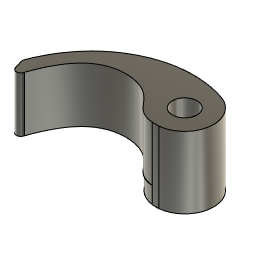
BarrelRatchet v3 (Autodesk Fusion 360 design; units mm, degrees)
Autodesk Fusion 360 part; units mm, degrees
sketch "base" plane through (0, 0, 0) normal (0, 0, 1) x (1, 0, 0)
  circle A0 centre (8.663, 2.8659) radius 2.25
  circle A1 centre (8.663, 2.8659) radius 5.25
  spline S0 degree 5 poles (-11.5756, -6.3241) (-11.5419, -6.2133) (-11.4706, -5.9871) (-11.3516, -5.634) (-11.1692, -5.1354) (-10.9008, -4.4671) (-10.591, -3.7572) (-10.2374, -3.0131) (-9.8371, -2.2479) (-9.3859, -1.4787) (-8.8802, -0.7244) (-8.3164, -0.0047) (-7.6922, 0.6618) (-7.007, 1.2599) (-6.2619, 1.777) (-5.4599, 2.2034) (-4.6063, 2.5325) (-3.7086, 2.7602) (-2.7767, 2.8854) (-1.823, 2.9086) (-0.8622, 2.8297) (0.0889, 2.6468) (1.0114, 2.3552) (1.8835, 1.9433) (2.6869, 1.4021) (3.4132, 0.7352) (4.0764, -0.0226) (4.711, -0.8083) (5.4062, -1.479) (6.2073, -1.9622) (7.1161, -2.254) (7.915, -2.3562) (8.5435, -2.3764) (8.9737, -2.3675) (9.1917, -2.3574) knots 0 0 0 0 0 0 0.033333 0.066667 0.1 0.133333 0.166667 0.2 0.233333 0.266667 0.3 0.333333 0.366667 0.4 0.433333 0.466667 0.5 0.533333 0.566667 0.6 0.633333 0.666667 0.7 0.733333 0.766667 0.8 0.833333 0.866667 0.9 0.933333 0.966667 1 1 1 1 1 1
  line L0 (2.9298, 1.2447) -> (6.1452, -2.3895)
  line L1 (6.5259, -2.4803) -> (11.8575, -2.2346)
  spline S1 degree 5 poles (-13.0568, -6.2405) (-13.083, -6.1478) (-13.1341, -5.9688) (-13.2069, -5.7196) (-13.2964, -5.4258) (-13.3947, -5.1212) (-13.4763, -4.8739) (-13.535, -4.6734) (-13.5618, -4.5011) (-13.547, -4.3234) (-13.4818, -4.0931) (-13.3607, -3.7703) (-13.1844, -3.3445) (-12.9588, -2.8306) (-12.6925, -2.257) (-12.3948, -1.6567) (-12.0736, -1.0557) (-11.7337, -0.4676) (-11.3776, 0.1025) (-11.0055, 0.6559) (-10.6157, 1.1973) (-10.2049, 1.7326) (-9.768, 2.2658) (-9.2993, 2.799) (-8.793, 3.3327) (-8.2438, 3.8659) (-7.6478, 4.396) (-7.0031, 4.9194) (-6.3106, 5.4309) (-5.5734, 5.9249) (-4.7961, 6.3952) (-3.9845, 6.8357) (-3.1451, 7.2405) (-2.2844, 7.6046) (-1.4083, 7.9242) (-0.5221, 8.1969) (0.3701, 8.4217) (1.2648, 8.5984) (2.1593, 8.7279) (3.0513, 8.8112) (3.9392, 8.8499) (4.8217, 8.8454) (5.6978, 8.7988) (6.567, 8.7112) (7.4288, 8.5833) (8.283, 8.4155) (8.9602, 8.2496) (9.4646, 8.1074) (9.7994, 8.0048) (9.9664, 7.9515) knots 0 0 0 0 0 0 0.022222 0.044444 0.066667 0.088889 0.111111 0.133333 0.155556 0.177778 0.2 0.222222 0.244444 0.266667 0.288889 0.311111 0.333333 0.355556 0.377778 0.4 0.422222 0.444444 0.466667 0.488889 0.511111 0.533333 0.555556 0.577778 0.6 0.622222 0.644444 0.666667 0.688889 0.711111 0.733333 0.755556 0.777778 0.8 0.822222 0.844444 0.866667 0.888889 0.911111 0.933333 0.955556 0.977778 1 1 1 1 1 1
  arc A2 (-13.0568, -6.2405) -> (-11.5103, -6.1151) centre (-12.2993, -5.9832) ccw
  point P0 (-10.553, -3.6897)
  point P1 (-8.28, 0.0068)
  point P2 (-4.5146, 2.5324)
  point P3 (0.3976, 2.5324)
  point P4 (4.5375, -0.5724)
  point P5 (-13.4234, -5.034)
  point P6 (-13.5492, -4.5396)
  point P7 (-13.4459, -4.0063)
  point P8 (-12.4929, -1.8607)
  point P9 (-10.5689, 1.2515)
  point P10 (-7.6643, 4.3699)
  point P11 (-2.2966, 7.5872)
  point P12 (4.0429, 8.8408)
  dimension "d1" = 4.5
  dimension "d2" = 10.5
  dimension "d3" = 1.6
  constraint concentric A0 A1
  constraint coincident S0.start A2
  constraint midpoint P4 L0
  constraint coincident A1 S0.end
  constraint midpoint S0.end L1
  constraint coincident A1 S1.end
  constraint coincident S0 A2.end
  measures "d1" diameter of A0
  measures "d2" diameter of A1
  measures "d3" diameter of A2
extrude "Extrude1" add sketch "base" against normal blind 3 contours A1 S0
extrude "Extrude2" add sketch "base" along normal blind 10 contours A1 S0 S1 A2
sketch "ring" plane through (0, 0, 0) normal (0, 0, 1) x (-1, 0, 0)
  circle A0 centre (-8.663, -2.8659) radius 2.25
  arc A1 (-9.1917, 2.3574) -> (-9.9664, -7.9515) centre (-8.663, -2.8659) ccw
  arc A2 (-9.9664, -7.9515) -> (-7.9665, 2.3377) centre (-8.663, -2.8659) ccw
  spline S0 degree 5 poles (-7.9665, 2.3377) (-7.9993, 2.3406) (-8.2364, 2.3599) (-8.4781, 2.3703) (-8.724, 2.3726) (-8.9737, 2.3675) (-9.1917, 2.3574) knots 0.961311 0.961311 0.961311 0.961311 0.961311 0.961311 0.966667 1 1 1 1 1 1
extrude "Extrude3" add sketch "ring" along normal blind 10
named bodies: "BarrelRatchet"
